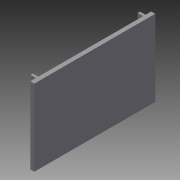
# Autodesk Inventor part: 40mm Side v1
Saved by Autodesk Inventor 2015 (Build 190159000, 159)
## iProperties
Created: 2018-01-01
Part Number: 40mm Side v1
Material: Generic
Document SubType Name: Modeling
Designer: Toby
Density: 1 g/cm^3
Appearance: Default
Author: Toby
Autodesk Inventor part; units mm, degrees
ref_plane "YZ Plane" through (0, 0, 0) normal (1, 0, 0) x (0, 1, 0)
ref_plane "XZ Plane" through (0, 0, 0) normal (0, 1, 0) x (-1, 0, 0)
ref_plane "XY Plane" through (0, 0, 0) normal (0, 0, 1) x (1, 0, 0)
sketch "Sketch1" plane through (0, 0, 0) normal (0, 0, 1) x (1, 0, 0)
  line L0 (-49.56, 19.825) -> (-47.46, 19.825)
  line L1 (-47.46, 19.825) -> (-47.46, -35.175)
  line L2 (-47.46, -35.175) -> (-49.56, -35.175)
  line L3 (-49.56, -35.175) -> (-49.56, 19.825)
  point P0 (0, 0)
  dimension "d0" = 2.1
  dimension "d1" = 55
  constraints: 8 end point, 2 parallel, 1 horizontal, 1 perpendicular
  measures "d0" distance between parallel lines of L3 L1
  measures "d1" distance of L2.end L0.start
extrude "Extrusion1" add sketch "Sketch1" along normal blind 40
sketch "Sketch2" plane through (-47.46, -35.175, 0) normal (1, 0, 0) x (0, 0, -1)
  line L0 (-40, 55) -> (0, 55)
  line L1 (0, 55) -> (0, 56.2)
  line L2 (0, 56.2) -> (-40, 56.2)
  line L3 (-40, 56.2) -> (-40, 55)
  line L4 (0, 0) -> (-40, 0)
  line L5 (-40, 0) -> (-40, -1.2)
  line L6 (-40, -1.2) -> (0, -1.2)
  line L7 (0, -1.2) -> (0, 0)
  line L8 (0, 55) -> (0, 0) projected
  line L9 (-40, 0) -> (-40, 55) projected
  point P0 (0, 35.175)
  dimension "d4" = 1.2
  dimension "d5" = 1.2
  constraints: 16 end point, 4 parallel, 2 collinear, 2 horizontal, 2 perpendicular
  measures "d4" distance between parallel lines of L0 L2
  measures "d5" distance between parallel lines of L6 L4
extrude "Extrusion2" add sketch "Sketch2" against normal blind 5 contours L3 L2 L1 L0 | L4 L7 L6 L5
sketch "Sketch3" plane through (-47.46, 21.025, 40) normal (0, 1, 0) x (1, 0, 0)
  line L0 (0, 40) -> (-2.1, 40)
  line L1 (-2.1, 40) -> (-2.1, 0)
  line L2 (-2.1, 0) -> (0, 0)
  line L3 (0, 0) -> (0, 40)
  point P0 (47.46, 40)
  constraints: 8 end point, 2 parallel, 1 horizontal, 1 perpendicular
extrude "Extrusion3" add sketch "Sketch3" along normal blind 3
sketch "Sketch4" plane through (-47.46, -36.375, 0) normal (0, -1, 0) x (1, 0, 0)
  line L0 (0, 40) -> (-2.1, 40)
  line L1 (-2.1, 40) -> (-2.1, 0)
  line L2 (-2.1, 0) -> (0, 0)
  line L3 (0, 0) -> (0, 40)
  point P0 (47.46, 0)
  constraints: 8 end point, 2 parallel, 1 horizontal, 1 perpendicular
extrude "Extrusion4" add sketch "Sketch4" along normal blind 3
body "Solid1"
